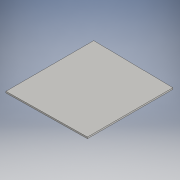
# Autodesk Inventor part: PlywoodForBed
Saved by Autodesk Inventor 2016 (Build 200138000, 138)
## iProperties
Created: 2015-10-19
Part Number: PlywoodForBed
Material: Generic
Document SubType Name: Modeling
Designer: steele
Density: 1 g/cm^3
Appearance: Default
Author: steele
Autodesk Inventor part; units mm, degrees
ref_plane "YZ Plane" through (0, 0, 0) normal (1, 0, 0) x (0, 1, 0)
ref_plane "XZ Plane" through (0, 0, 0) normal (0, 1, 0) x (-1, 0, 0)
ref_plane "XY Plane" through (0, 0, 0) normal (0, 0, 1) x (1, 0, 0)
sketch "Sketch1" plane through (0, 0, 0) normal (0, 1, 0) x (-1, 0, 0)
  line L0 (0, 0) -> (0, -904.875)
  line L1 (0, 0) -> (850.9, 12.3825)
  line L2 (0, -904.875) -> (850.9, -917.2575)
  line L3 (850.9, -917.2575) -> (850.9, 12.3825)
  line L4 (0, 0) -> (850.9, 0) construction
  line L5 (0, -904.875) -> (850.9, -904.875) construction
  line L6 (425.45, 6.1912) -> (425.45, -911.0663)
  dimension "d0" = 904.875
  dimension "d1" = 929.64
  dimension "d2" = 850.9
  dimension "d3" = 425.45
  constraints: 14 end point, 3 perpendicular, 2 midpoint, 2 point on line, 2 vertical, 1 equal length
  measures "d0" distance of L0.start L0.end
  measures "d1" distance of L2.end L1.end
  measures "d2" distance between parallel lines of L0 L3
  measures "d3" distance between parallel lines of L6 L0
extrude "Extrusion1" add sketch "Sketch1" along normal blind 15.875
body "Solid1"
